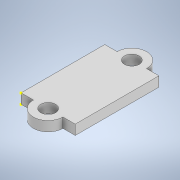
# Autodesk Inventor part: przykrywka
Saved by Autodesk Inventor 2020.5 (Build 245400000, 400)
## iProperties
Created: 2023-04-01
Part Number: przykrywka
Material: Generic
Document SubType Name: Modeling
Designer: aniela
Density: 1 g/cm^3
Appearance: Default
Author: aniela
Autodesk Inventor part; units mm, degrees
ref_plane "YZ Plane" through (0, 0, 0) normal (1, 0, 0) x (0, 1, 0)
ref_plane "XZ Plane" through (0, 0, 0) normal (0, 1, 0) x (-1, 0, 0)
ref_plane "XY Plane" through (0, 0, 0) normal (0, 0, 1) x (1, 0, 0)
sketch "Sketch1" plane through (0, 0, 0) normal (0, 1, 0) x (-1, 0, 0)
  line L0 (0, 0) -> (-11, 0)
  line L1 (-11, 0) -> (-11, -17)
  line L2 (-11, -17) -> (0, -17)
  line L3 (0, -17) -> (0, 0)
  circle A0 centre (-5.5, 0) radius 3
  circle A1 centre (-5.5, -17) radius 3
  circle A2 centre (-5.5, 0) radius 1.5
  circle A3 centre (-5.5, -17) radius 1.5
  circle A4 centre (-5.5, -17) radius 3
  circle A5 centre (-5.5, -17) radius 1.5
  circle A6 centre (-5.5, 0) radius 1.5
  circle A7 centre (-5.5, 0) radius 3
  point P0 (-8.5, -17)
  point P1 (-2.5, -17)
  point P2 (-2.5, 0)
  point P3 (-8.5, 0)
  dimension "d0" = 11
  dimension "d1" = 17
  dimension "d2" = 6
  dimension "d3" = 6
  dimension "d6" = 3
  dimension "d7" = 3
  constraints: 8 centre point, 8 end point, 6 coincident, 4 concentric, 2 midpoint, 2 parallel, 1 horizontal, 1 perpendicular
  measures "d0" distance of L2.end L1.end
  measures "d1" distance of L1.end L0.end
  measures "d2" diameter of A0
  measures "d3" diameter of A1
  measures "d6" diameter of A2
  measures "d7" diameter of A3
extrude "Extrusion1" add sketch "Sketch1" along normal blind 2
sketch "Sketch2" plane through (0, 2, 0) normal (0, 1, 0) x (1, 0, 0)
  point P0 (0, 0)
sketch "Sketch3" plane through (0, 0, 0) normal (0, -1, 0) x (1, 0, 0)
  point P0 (0, 0)
sketch "Sketch4" plane through (0, 0, 0) normal (0, -1, 0) x (1, 0, 0)
  arc A0 (8.5, 0) -> (2.5, 0) centre (5.5, 0) ccw projected
  circle A1 centre (5.5, 0) radius 1.5
  arc A2 (2.5, -17) -> (8.5, -17) centre (5.5, -17) ccw projected
  circle A3 centre (5.5, -17) radius 1.5
  circle A4 centre (5.5, -17) radius 1.5
  circle A5 centre (5.5, 0) radius 1.5
  point P0 (0, 0)
  dimension "d8" = 3
  dimension "d9" = 3
  constraints: 4 centre point, 4 coincident, 2 concentric
  measures "d8" diameter of A1
  measures "d9" diameter of A3
hole "Hole1" at (5.5, 0, 0) at (5.5, 0, -17) direction (0, 1, 0) diameter 3 end through all
body "Solid1"
